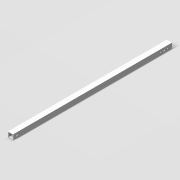
# Autodesk Inventor part: custom Box Aluminum
Saved by Autodesk Inventor 2013 (Build 170138000, 138)
## iProperties
Created: 2013-12-23
Part Number: custom Box Aluminum
Material: Aluminum 6061
Document SubType Name: Modeling
Designer: kahohbein
Density: 1 g/cm^3
Author: kahohbein
Autodesk Inventor part; units mm, degrees
ref_plane "YZ Plane" through (0, 0, 0) normal (1, 0, 0) x (0, 1, 0)
ref_plane "XZ Plane" through (0, 0, 0) normal (0, 1, 0) x (-1, 0, 0)
ref_plane "XY Plane" through (0, 0, 0) normal (0, 0, 1) x (1, 0, 0)
sketch "Sketch1" plane through (0, 0, 0) normal (0, 0, 1) x (1, 0, 0)
  line L0 (0, 0) -> (12.5476, 0)
  line L1 (12.5476, 0) -> (12.5476, 12.5476)
  line L2 (12.5476, 12.5476) -> (0, 12.5476)
  line L3 (0, 12.5476) -> (0, 0)
  line L4 (1.5113, 1.5113) -> (11.0363, 1.5113)
  line L5 (11.0363, 1.5113) -> (11.0363, 11.0363)
  line L6 (11.0363, 11.0363) -> (1.5113, 11.0363)
  line L7 (1.5113, 11.0363) -> (1.5113, 1.5113)
  line L8 (1.5113, 1.5113) -> (11.0363, 11.0363) construction
  line L9 (11.0363, 1.5113) -> (1.5113, 11.0363) construction
  point P0 (6.2738, 6.2738)
  dimension "d0" = 12.5476
  dimension "d1" = 12.5476
  dimension "d2" = 9.525
  dimension "d3" = 9.525
  constraints: 20 end point, 4 parallel, 2 horizontal, 2 midpoint, 2 perpendicular
  measures "d0" distance of L2.end L1.end
  measures "d1" distance of L1.end L0.end
  measures "d2" distance of L6.end L5.end
  measures "d3" distance of L5.end L4.end
extrude "Extrusion1" add sketch "Sketch1" along normal blind 381
sketch "Sketch2" plane through (12.5476, 0, 0) normal (1, 0, 0) x (0, 0, -1)
  circle A0 centre (-19.05, 6.2738) radius 2.413
  line L0 (0, 0) -> (0, 12.5476) projected
  dimension "d6" = 4.826
  dimension "d13" = 19.05
  constraints: 1 centre point
  measures "d6" diameter of A0
  measures "d13" distance from line of L0 A0.centre
extrude "Extrusion2" cut sketch "Sketch2" against normal blind 419.1
sketch "Sketch3" plane through (12.5476, 0, 0) normal (1, 0, 0) x (0, 0, -1)
  circle A0 centre (-372.11, 6.2738) radius 2.413
  line L0 (-381, 0) -> (-381, 12.5476) projected
  dimension "d9" = 4.826
  dimension "d12" = 8.89
  constraints: 1 centre point
  measures "d9" diameter of A0
  measures "d12" distance from line of L0 A0.centre
extrude "Extrusion3" cut sketch "Sketch3" against normal blind 25.4
sketch "Sketch5" plane through (0, 0, 0) normal (-1, 0, 0) x (0, 0, 1)
  circle A0 centre (19.05, 6.2738) radius 2.413 projected
  circle A1 centre (11.05, 6.2738) radius 1.3462
  circle A2 centre (27.05, 6.2738) radius 1.3462
  line L0 (0, 12.5476) -> (381, 12.5476) projected
  line L1 (11.05, 6.2738) -> (27.05, 6.2738)
  line L2 (0, 12.5476) -> (0, 0) projected
  dimension "d14" = 2.6924
  dimension "d15" = 2.6924
  dimension "d16" = 16
  dimension "d19" = 11.05
  dimension "d20" = 19.05
  dimension "d21" = 27.05
  constraints: 2 centre point, 2 coincident, 2 end point, 1 midpoint, 1 parallel
  measures "d14" diameter of A1
  measures "d15" diameter of A2
  measures "d16" distance of L1.end L1.start
  measures "d19" distance from line of L2 L1.start
  measures "d20" distance from line of L2 A0.centre
  measures "d21" distance from line of L2 L1.end
extrude "Extrusion4" cut sketch "Sketch5" against normal blind 12.7 contours A1 | A2
body "Solid1"
